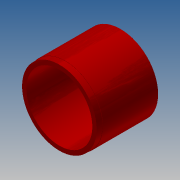
# Autodesk Inventor part: A1-19027-400-09 HCWI liner - drain
Saved by Autodesk Inventor 2017.3 (Build 213257000, 257)
## iProperties
Created: 2019-08-16
Part Number: A1-19027-400-09 HCWI liner - drain
Material: Iron, HCWI
Document SubType Name: Modeling
Designer: GVD
Density: 7.33517 g/cm^3
Appearance: Iron Gray(1)
Mass: 36761.9 g
Surface Area: 5383.38 cm^2
Volume: 5011.73 cm^3
Description: 11 1/8" ID x 13/16" WALL x 10 11/32" HCWI LINER, ASTM A532 CLASS III TYPE A, PF# 470297
Author: GVD
Autodesk Inventor part; units mm, degrees
ref_plane "YZ Plane" through (0, 0, 0) normal (1, 0, 0) x (0, 1, 0)
ref_plane "XZ Plane" through (0, 0, 0) normal (0, 1, 0) x (-1, 0, 0)
ref_plane "XY Plane" through (0, 0, 0) normal (0, 0, 1) x (1, 0, 0)
sketch "Sketch1" plane through (0, 0, 0) normal (0, 0, 1) x (1, 0, 0)
  circle A0 centre (0, 0) radius 141.5
  circle A1 centre (0, 0) radius 161.671
  dimension "d0" = 283
  dimension "d1" = 323.342
  constraints: 2 centre point, 2 coincident
  measures "d0" diameter of A0
  measures "d1" diameter of A1
extrude "Extrusion1" add sketch "Sketch1" along normal blind 263
sketch "Sketch2" plane through (0, 0, 263) normal (0, 0, 1) x (1, 0, 0)
  circle A0 centre (0, 0) radius 161.671 projected
  circle A1 centre (0, 0) radius 160.0835
  dimension "d4" = 320.167
  constraints: 1 centre point, 1 coincident
  measures "d4" diameter of A1
extrude "Extrusion2" cut sketch "Sketch2" against normal blind 25.4
fillet "Fillet1" radius 0.7937 1 edges at (-160.0835, 0, 237.6)
chamfer "Chamfer1" distance 0.7937 angle 45 1 edges at (-161.671, 0, 0)
body "Solid1"
